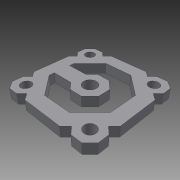
# Autodesk Inventor part: x_iddler_belt_bearing_mount
Saved by Autodesk Inventor 2014 (Build 180170000, 170)
## iProperties
Created: 2013-12-02
Part Number: x_iddler_belt_bearing_mount
Material: Generic
Document SubType Name: Modeling
Designer: buben
Density: 1 g/cm^3
Appearance: Anodized - Dark Gray
Author: buben
Subject: Laser Cutted
Autodesk Inventor part; units mm, degrees
ref_plane "YZ Plane" through (0, 0, 0) normal (1, 0, 0) x (0, 1, 0)
ref_plane "XZ Plane" through (0, 0, 0) normal (0, 1, 0) x (-1, 0, 0)
ref_plane "XY Plane" through (0, 0, 0) normal (0, 0, 1) x (1, 0, 0)
sketch "Sketch1" plane through (0, 0, 0) normal (0, 0, 1) x (1, 0, 0)
  circle A0 centre (0, 0) radius 8 construction
  circle A1 centre (0, 0) radius 16 construction
  line L0 (20, -8.2843) -> (8.2843, -20)
  line L1 (8.2843, -20) -> (-8.2843, -20)
  line L2 (-8.2843, -20) -> (-20, -8.2843)
  line L3 (-20, 8.2843) -> (-8.2843, 20)
  line L4 (-8.2843, 20) -> (8.2843, 20)
  line L5 (8.2843, 20) -> (20, 8.2843)
  line L6 (20, 8.2843) -> (20, -8.2843)
  line L7 (-7.7279, 5) -> (-20, 5)
  line L8 (-7.7279, -5) -> (-20, -5)
  circle A2 centre (0, 0) radius 4.2
  line L9 (-20, -8.2843) -> (-20, -5)
  line L10 (-20, 5) -> (-20, 8.2843)
  line L11 (28, -11.598) -> (11.598, -28)
  line L12 (11.598, -28) -> (-11.598, -28)
  line L13 (-11.598, -28) -> (-28, -11.598)
  line L14 (-28, -11.598) -> (-28, 11.598)
  line L15 (-28, 11.598) -> (-11.598, 28)
  line L16 (-11.598, 28) -> (11.598, 28)
  line L17 (11.598, 28) -> (28, 11.598)
  line L18 (28, 11.598) -> (28, -11.598)
  line L19 (9, -3.7279) -> (3.7279, -9)
  line L20 (3.7279, -9) -> (-3.7279, -9)
  line L21 (-3.7279, 9) -> (3.7279, 9)
  line L22 (3.7279, 9) -> (9, 3.7279)
  line L23 (9, 3.7279) -> (9, -3.7279)
  line L24 (-20, 5) -> (-20, -5) construction
  line L25 (-3.7279, 9) -> (-7.7279, 5)
  line L26 (-3.7279, -9) -> (-7.7279, -5)
  point P0 (-20, 0)
  dimension "d1" = 16
  dimension "d2" = 32
  dimension "d5" = 8.4
  dimension "d6" = 40
  dimension "d7" = 8
  dimension "d8" = 10
  dimension "d10" = 18
  constraints: 54 end point, 6 coincident, 6 perpendicular, 3 centre point, 2 horizontal alignment, 1 collinear, 1 midpoint, 1 parallel, 42 other
  measures "d1" diameter of A0
  measures "d2" diameter of A1
  measures "d5" diameter of A2
  measures "d6" distance between parallel lines of L6 L9
  measures "d7" distance between parallel lines of L14 L9
  measures "d8" distance between parallel lines of L7 L8
  measures "d10" distance between parallel lines of L21 L20
extrude "Extrusion1" add sketch "Sketch1" along normal blind 6
sketch "Sketch2" plane through (0, 0, 6) normal (0, 0, 1) x (1, 0, 0)
  circle A0 centre (0, 0) radius 4.2 projected
  line L0 (11.598, 28) -> (-11.598, 28) projected
  line L1 (-11.598, 28) -> (-28, 11.598) projected
  line L2 (-28, 11.598) -> (-28, -11.598) projected
  line L3 (-28, -11.598) -> (-11.598, -28) projected
  line L4 (-11.598, -28) -> (11.598, -28) projected
  line L5 (-24.7487, 14.8492) -> (-28, 18.1005)
  line L6 (-28, 18.1005) -> (-28, 23.8995)
  line L7 (-28, 23.8995) -> (-23.8995, 28)
  line L8 (-23.8995, 28) -> (-18.1005, 28)
  line L9 (-18.1005, 28) -> (-14.8492, 24.7487)
  line L10 (-28, 21) -> (-21, 21) construction
  line L11 (-21, 28) -> (-21, 21) construction
  circle A1 centre (-21, 21) radius 3.2
  line L12 (-24.7487, 14.8492) -> (-14.8492, 24.7487)
  line L13 (-14.8492, -24.7487) -> (-18.1005, -28)
  line L14 (-18.1005, -28) -> (-23.8995, -28)
  line L15 (-23.8995, -28) -> (-28, -23.8995)
  line L16 (-28, -23.8995) -> (-28, -18.1005)
  line L17 (-28, -18.1005) -> (-24.7487, -14.8492)
  circle A2 centre (-21, -21) radius 3.2
  line L18 (-14.8492, -24.7487) -> (-24.7487, -14.8492)
  line L19 (24.7487, -14.8492) -> (28, -18.1005)
  line L20 (28, -18.1005) -> (28, -23.8995)
  line L21 (28, -23.8995) -> (23.8995, -28)
  line L22 (23.8995, -28) -> (18.1005, -28)
  line L23 (18.1005, -28) -> (14.8492, -24.7487)
  circle A3 centre (21, -21) radius 3.2
  line L24 (24.7487, -14.8492) -> (14.8492, -24.7487)
  line L25 (14.8492, 24.7487) -> (18.1005, 28)
  line L26 (18.1005, 28) -> (23.8995, 28)
  line L27 (23.8995, 28) -> (28, 23.8995)
  line L28 (28, 23.8995) -> (28, 18.1005)
  line L29 (28, 18.1005) -> (24.7487, 14.8492)
  circle A4 centre (21, 21) radius 3.2
  line L30 (14.8492, 24.7487) -> (24.7487, 14.8492)
  circle A5 centre (-21, 21) radius 6 construction
  point P0 (-19.799, 19.799)
  point P1 (-21, -28)
  point P2 (-28, -21)
  point P3 (28, -21)
  point P4 (21, -28)
  point P5 (21, 28)
  point P6 (28, 21)
  dimension "d13" = 14
  dimension "d14" = 7
  dimension "d15" = 6.4
  dimension "d18" = 360
  dimension "d22" = 12
  constraints: 52 end point, 6 perpendicular, 5 centre point, 3 midpoint, 2 coincident, 2 collinear, 2 parallel, 2 point on line, 1 equal length, 65 other
  measures "d13" distance between parallel lines of L9 L5
  measures "d14" distance from line of point (-19.799, 19.799) L5
  measures "d15" diameter of A1
  measures "d22" diameter of A5
extrude "Extrusion2" add sketch "Sketch2" against normal blind 6 contours L3 A2 L13 L14 L15 L16 L17 | L5 L6 L7 L8 L9 L1 A1 | L19 L20 L21 L22 L23 L24 A3 | L25 L26 L27 L28 L29 L30 A4
sketch "Sketch3" plane through (0, 0, 6) normal (0, 0, 1) x (1, 0, 0)
  line L0 (-17.8813, 21.7167) -> (-21.7167, 17.8813) projected
  arc A0 (-17.8813, 21.7167) -> (-21.7167, 17.8813) centre (-21, 21) ccw projected
  line L1 (-21.7167, -17.8813) -> (-17.8813, -21.7167) projected
  arc A1 (-21.7167, -17.8813) -> (-17.8813, -21.7167) centre (-21, -21) ccw projected
  arc A2 (17.8813, -21.7167) -> (21.7167, -17.8813) centre (21, -21) ccw projected
  line L2 (17.8813, -21.7167) -> (21.7167, -17.8813) projected
  arc A3 (21.7167, 17.8813) -> (17.8813, 21.7167) centre (21, 21) ccw projected
  line L3 (21.7167, 17.8813) -> (17.8813, 21.7167) projected
  circle A4 centre (-21, -21) radius 3.2
  circle A5 centre (-21, 21) radius 3.2
  circle A6 centre (21, 21) radius 3.2
  circle A7 centre (21, -21) radius 3.2
  constraints: 4 coincident, 12 other
extrude "Extrusion3" cut sketch "Sketch3" against normal through all contours A5 L0 | A4 L1 | A7 L2 | A6 L3
body "Solid1"
